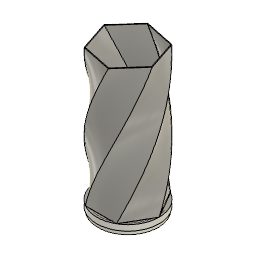
Assembly_lamp (Autodesk Fusion 360 archive; units mm, degrees)
design "hull_twisted"
part number: 2026-05-21-14-33-30-089
Autodesk Fusion 360 part; units mm, degrees
sketch "Sketch1" plane through (0, 0, 0) normal (0, 0, 1) x (1, 0, 0)
  circle A0 centre (0, 0) radius 38.75
  circle A1 centre (0, 0) radius 36.95
  dimension "d1" = 77.5
  dimension "d2" = 73.9
  constraint coincident A0.centre A1.centre
  constraint concentric A0 A1
  measures "d1" diameter of A0
  measures "d2" diameter of A1
extrude "Extrude1" add sketch "Sketch1" along normal blind 4.8 from surface at 17.9
sketch "Sketch2" plane through (0, 0, 22.7) normal (0, 0, 1) x (-1, 0, 0)
  circle A0 centre (0, 0) radius 36.95
  circle A1 centre (0, 0) radius 38.75
  circle A2 centre (0, 0) radius 40
  dimension "d6" = 80
  constraint coincident A0.centre A1.centre
  measures "d6" diameter of A2
extrude "Extrude2" add sketch "Sketch2" along normal blind 7.3 contours A1 | A2
sketch "Sketch3" plane through (0, 0, 30) normal (0, 0, 1) x (-1, 0, 0)
  circle A0 centre (0, 0) radius 36.95
  circle A1 centre (0, 0) radius 40
  line L0 (-20, 34.641) -> (-40, 0)
  line L1 (-40, 0) -> (-20, -34.641)
  line L2 (-20, -34.641) -> (20, -34.641)
  line L3 (20, -34.641) -> (40, 0)
  line L4 (40, 0) -> (20, 34.641)
  line L5 (20, 34.641) -> (-20, 34.641)
  line L6 (38.8453, 0) -> (19.4226, 33.641)
  line L7 (19.4226, 33.641) -> (-19.4226, 33.641)
  line L8 (-19.4226, 33.641) -> (-38.8453, 0)
  line L9 (-38.8453, 0) -> (-19.4226, -33.641)
  line L10 (-19.4226, -33.641) -> (19.4226, -33.641)
  line L11 (19.4226, -33.641) -> (38.8453, 0)
  dimension "d9" = 40
  dimension "d10" = -1
  constraint coincident A0.centre A1.centre
  constraint horizontal L3.end A0.centre
  measures "d9" distance of L0.start A0.centre
sketch "Sketch4" plane through (0, 0, 0) normal (0, 1, 0) x (1, 0, 0)
  line L0 (0, -30) -> (0, -200)
  dimension "d11" = 170
  constraint vertical L0
  measures "d11" distance of L0.start L0.end
sweep "Sweep1" add twist angle 108.3 profiles "Sketch3" path "Sketch4" along L0 section 1 contours A0 L4 L6 | A0 L3 L4 L6 L11 | A0 L3 L11 | A0 L4 L5 L6 L7 | A0 L2 L3 L10 L11 | A0 L5 L7 | A0 L2 L10 | A0 L0 L5 L7 L8 | A0 L1 L2 L9 L10 | A0 L0 L8 | A0 L1 L9 | A0 L0 L1 L8 L9
sketch "Sketch5" plane through (0, 0, 30) normal (0, 0, 1) x (-1, 0, 0)
  line L0 (-20, -34.641) -> (-23.5715, -28.455)
  arc A0 (-36.4285, -6.186) -> (-23.5715, -28.455) centre (0, 0) ccw
  line L1 (-36.4285, -6.186) -> (-40, 0)
  arc A1 (-40, 0) -> (-20, -34.641) centre (0, 0) ccw
  arc A2 (-36.4285, -6.186) -> (-23.5715, -28.455) centre (0, 0) ccw
  line L2 (-36.4285, -6.186) -> (-23.5715, -28.455)
extrude "Extrude3" add sketch "Sketch5" against normal blind 0.8 contours A0 A2 L2
pattern_circular "C-Pattern1" count 6 over 360 about axis through (0, 0, 1.75) along (0, 0, 1) of "Extrude3"

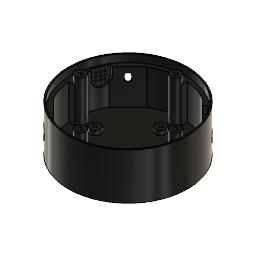
design "LAMP - BASE"
part number: 2026-05-21-10-57-22-259
Autodesk Fusion 360 part; units mm, degrees
sketch "Sketch1" plane through (0, 0, 0) normal (0, 0, 1) x (1, 0, 0)
  circle A0 centre (0, 0) radius 40
  circle A1 centre (0, 0) radius 39
  dimension "d1" = 80
  dimension "d2" = 78
  constraint coincident A0.centre A1.centre
  measures "d1" diameter of A0
  measures "d2" diameter of A1
extrude "Extrude1" add sketch "Sketch1" along normal blind 31
sketch "Sketch2" plane through (0, 0, 0) normal (0, 0, 1) x (1, 0, 0)
  circle A0 centre (0, 0) radius 39
  circle A1 centre (0, 0) radius 36.5
  dimension "d5" = 78
  dimension "d6" = 73
  constraint coincident A0.centre A1.centre
  constraint concentric A0 A1
  measures "d5" diameter of A0
  measures "d6" diameter of A1
extrude "Extrude2" add sketch "Sketch2" along normal blind 2.5 contours A0 | A1
extrude "Extrude3" add sketch "Sketch2" along normal blind 26
sketch "Sketch3" plane through (0, 0, 2.5) normal (0, 0, 1) x (-1, 0, 0)
  circle A0 centre (0, 0) radius 36.5
  circle A1 centre (0, 22) radius 3.5
  circle A2 centre (0, 22) radius 1.25
  circle A3 centre (-22, 0) radius 3.5
  circle A4 centre (-22, 0) radius 1.25
  circle A5 centre (0, -22) radius 3.5
  circle A6 centre (0, -22) radius 1.25
  circle A7 centre (22, 0) radius 3.5
  circle A8 centre (22, 0) radius 1.25
  dimension "d11" = 7
  dimension "d12" = 2.5
  dimension "d13" = 22
  dimension "d15" = 360
  constraint concentric A1 A2
  constraint vertical A0.centre A1.centre
  measures "d11" diameter of A1
  measures "d12" diameter of A2
  measures "d13" distance of A0.centre A1.centre
extrude "Extrude4" add sketch "Sketch3" along normal blind 3 contours A1 | A3 | A5 | A7
sketch "Sketch4" plane through (0, 0, 2.5) normal (0, 0, 1) x (-1, 0, 0)
  circle A0 centre (0, -22) radius 3.5
  circle A1 centre (-22, 0) radius 3.5
  circle A2 centre (0, 0) radius 36.5
  circle A3 centre (22, 0) radius 3.5
  circle A4 centre (0, 22) radius 3.5
  circle A5 centre (0, 32) radius 3.5
  circle A6 centre (0, 32) radius 1.25
  circle A7 centre (0, 0) radius 36.5
  line L0 (-3.5, 32) -> (-3.5, 36.3318)
  line L1 (3.5, 32) -> (3.5, 36.3318)
  dimension "d18" = 7
  dimension "d19" = 2.5
  dimension "d20" = 32
  constraint concentric A5 A6
  constraint vertical A2.centre A5.centre
  constraint coincident A5 L0.start
  constraint coincident A2 L0.end
  constraint tangent A5 L0
  constraint vertical L0
  constraint coincident A5 L1.start
  constraint coincident A2 L1.end
  constraint tangent A5 L1
  constraint parallel L0 L1
  measures "d18" diameter of A5
  measures "d19" diameter of A6
  measures "d20" vertical distance of A2.centre A5.centre
extrude "Extrude5" add sketch "Sketch4" along normal blind 28.5 contours A5
extrude "Extrude6" add sketch "Sketch4" along normal blind 23.5 contours A2 A5 A7 L0 L1 picked at (-2.1394, 35.9481)
pattern_circular "C-Pattern1" count 4 over 360 about axis through (0, 0, 1.75) along (0, 0, 1) of "Extrude5", "Extrude6"
sketch "Sketch5" plane through (0, 0, 26) normal (0, 0, 1) x (-1, 0, 0)
  arc A0 (36.3318, 3.5) -> (3.5, 36.3318) centre (0, 0) ccw
  circle A1 centre (0, 0) radius 39
  arc A2 (3.5, -36.3318) -> (36.3318, -3.5) centre (0, 0) ccw
  arc A3 (-36.3318, -3.5) -> (-3.5, -36.3318) centre (0, 0) ccw
  arc A4 (-3.5, 36.3318) -> (-36.3318, 3.5) centre (0, 0) ccw
  arc A5 (36.3318, 3.5) -> (3.5, 36.3318) centre (0, 0) ccw
  line L0 (31.3167, -18.7487) -> (18.7432, -31.32)
  line L1 (0, 0) -> (0, -13.7257) construction
  line L2 (0, 0) -> (13.0082, 0) construction
  line L3 (-31.3167, -18.7487) -> (-18.7432, -31.32)
  line L4 (31.3167, 18.7487) -> (18.7432, 31.32)
  line L5 (36.3318, 3.5) -> (32, 3.5)
  arc A6 (32, -3.5) -> (32, 3.5) centre (32, 0) ccw
  line L6 (32, -3.5) -> (36.3318, -3.5)
  arc A7 (3.5, -36.3318) -> (36.3318, -3.5) centre (0, 0) ccw
  line L7 (3.5, -36.3318) -> (3.5, -32)
  arc A8 (-3.5, -32) -> (3.5, -32) centre (0, -32) ccw
  line L8 (-3.5, -32) -> (-3.5, -36.3318)
  arc A9 (-36.3318, -3.5) -> (-3.5, -36.3318) centre (0, 0) ccw
  line L9 (-36.3318, -3.5) -> (-32, -3.5)
  arc A10 (-32, 3.5) -> (-32, -3.5) centre (-32, 0) ccw
  line L10 (-32, 3.5) -> (-36.3318, 3.5)
  arc A11 (-3.5, 36.3318) -> (-36.3318, 3.5) centre (0, 0) ccw
  line L11 (-3.5, 36.3318) -> (-3.5, 32)
  arc A12 (3.5, 32) -> (-3.5, 32) centre (0, 32) ccw
  line L12 (3.5, 32) -> (3.5, 36.3318)
  dimension "d27" = 17.78
  dimension "d28" = 16.046
  constraint coincident A0.centre A1.centre
  constraint vertical L1
  constraint perpendicular L1 L2
  constraint symmetric L0.start L1 L3.start
  constraint symmetric L0.end L1 L3.end
  constraint symmetric L0.start L2 L4.start
  constraint symmetric L0.end L2 L4.end
  measures "d27" distance of L0.start L0.end
  measures "d28" distance of A2.start L0.end
extrude "Extrude7" add sketch "Sketch5" against normal blind 23.5 contours A0 A5 L4 | A2 L0 A7 | A3 L3 A9
sketch "Sketch6" plane through (-25.03, -25.0344, 0) normal (0.707045, 0.707169, 0) x (-0.707169, 0.707045, 0)
  line L0 (-8.89, 2.5) -> (8.89, 2.5)
  line L1 (8.89, 2.5) -> (8.89, 26)
  line L2 (8.89, 26) -> (-8.89, 26)
  line L3 (-8.89, 26) -> (-8.89, 2.5)
  circle A0 centre (0, 13.5) radius 4.5
  dimension "d31" = 9
  dimension "d32" = 13.5
  constraint vertical origin A0.centre
  measures "d31" diameter of A0
  measures "d32" distance of origin A0.centre
extrude "Extrude8" cut sketch "Sketch6" against normal through all contours A0
sketch "Sketch7" plane through (-25.03, 25.0344, 0) normal (0.707045, -0.707169, 0) x (0.707169, 0.707045, 0)
  line L0 (-8.89, 2.5) -> (8.89, 2.5)
  line L1 (8.89, 2.5) -> (8.89, 26)
  line L2 (8.89, 26) -> (-8.89, 26)
  line L3 (-8.89, 26) -> (-8.89, 2.5)
  line L4 (-1.725, 21.025) -> (-1.725, 18.975)
  arc A0 (-1.725, 18.975) -> (1.725, 18.975) centre (0, 18.975) ccw
  line L5 (1.725, 18.975) -> (1.725, 21.025)
  arc A1 (1.725, 21.025) -> (-1.725, 21.025) centre (0, 21.025) ccw
  line L6 (0, 22.75) -> (0, 17.25) construction
  dimension "d34" = 3.45
  dimension "d35" = 5.5
  dimension "d36" = 14.75
  constraint tangent L4 A0
  constraint tangent A0 L5
  constraint parallel L4 L5
  constraint tangent L5 A1
  constraint tangent L4 A1
  constraint coincident A1 L6.start
  constraint coincident A0 L6.end
  constraint coincident A0.centre L6
  constraint coincident A1.centre L6
  constraint vertical L6
  constraint vertical origin A0.centre
  measures "d34" distance of L4 L5
  measures "d35" distance of L6.start L6.end
  measures "d36" distance of L0 L6.end
extrude "Extrude9" cut sketch "Sketch7" against normal blind 0.698 contours L4 A0 L5 A1
extrude "Extrude10" cut sketch "Sketch7" against normal through all draft 37 from surface at -0.698 contours L4 A0 L5 A1
sketch "Sketch8" plane through (25.03, 25.0344, 0) normal (-0.707045, -0.707169, 0) x (0.707169, -0.707045, 0)
  line L0 (8.89, 26) -> (-8.89, 26)
  line L1 (-8.89, 26) -> (-8.89, 2.5)
  line L2 (-8.89, 2.5) -> (8.89, 2.5)
  line L3 (8.89, 2.5) -> (8.89, 26)
  circle A0 centre (0, 11) radius 3.5
  line L4 (-3.5, 26) -> (-3.5, 11)
  line L5 (3.5, 26) -> (3.5, 11)
  dimension "d41" = 7
  dimension "d42" = 11
  constraint vertical origin A0.centre
  constraint coincident L0 L4.start
  constraint perpendicular L0 L4
  constraint coincident L0 L5.start
  constraint coincident A0 L5.end
  constraint coincident A0 L4.end
  constraint tangent A0 L4
  constraint tangent A0 L5
  constraint vertical L5
  measures "d41" diameter of A0
  measures "d42" vertical distance of origin A0.centre
extrude "Extrude11" cut sketch "Sketch8" against normal blind 2.6 contours L0 A0 L4 L5 | A0
extrude "Extrude12" cut sketch "Sketch8" against normal blind 4.6 contours A0
sketch "Sketch9" plane through (0, 0, 26) normal (0, 0, 1) x (-1, 0, 0)
  circle A0 centre (0, 0) radius 39
  line L0 (-22.5549, -27.509) -> (-24.3932, -29.3477)
  line L1 (-24.3932, -29.3477) -> (-29.3434, -24.3983)
  line L2 (-29.3434, -24.3983) -> (-27.505, -22.5597)
  line L3 (-27.505, -22.5597) -> (-31.3167, -18.7487)
  arc A1 (-36.3318, -3.5) -> (-31.3167, -18.7487) centre (0, 0) ccw
  line L4 (-36.3318, -3.5) -> (-32, -3.5)
  arc A2 (-32, 3.5) -> (-32, -3.5) centre (-32, 0) ccw
  line L5 (-32, 3.5) -> (-36.3318, 3.5)
  arc A3 (-3.5, 36.3318) -> (-36.3318, 3.5) centre (0, 0) ccw
  line L6 (-3.5, 36.3318) -> (-3.5, 32)
  arc A4 (3.5, 32) -> (-3.5, 32) centre (0, 32) ccw
  line L7 (3.5, 32) -> (3.5, 36.3318)
  arc A5 (18.7432, 31.32) -> (3.5, 36.3318) centre (0, 0) ccw
  line L8 (18.7432, 31.32) -> (31.3167, 18.7487)
  arc A6 (36.3318, 3.5) -> (31.3167, 18.7487) centre (0, 0) ccw
  line L9 (36.3318, 3.5) -> (32, 3.5)
  arc A7 (32, -3.5) -> (32, 3.5) centre (32, 0) ccw
  line L10 (32, -3.5) -> (36.3318, -3.5)
  arc A8 (31.3167, -18.7487) -> (36.3318, -3.5) centre (0, 0) ccw
  line L11 (31.3167, -18.7487) -> (18.7432, -31.32)
  arc A9 (3.5, -36.3318) -> (18.7432, -31.32) centre (0, 0) ccw
  line L12 (3.5, -36.3318) -> (3.5, -32)
  arc A10 (-3.5, -32) -> (3.5, -32) centre (0, -32) ccw
  line L13 (-3.5, -32) -> (-3.5, -36.3318)
  arc A11 (-18.7432, -31.32) -> (-3.5, -36.3318) centre (0, 0) ccw
  line L14 (-18.7432, -31.32) -> (-22.5549, -27.509)
  line L15 (31.3167, -18.7487) -> (18.7432, -31.32)
  arc A12 (31.3167, -18.7487) -> (36.3318, -3.5) centre (0, 0) ccw
  arc A13 (3.5, -36.3318) -> (18.7432, -31.32) centre (0, 0) ccw
  line L16 (36.4457, -10.9357) -> (32.1385, -20.5117)
  line L17 (32.1385, -20.5117) -> (30.3555, -19.7097)
  line L18 (36.4457, -10.9357) -> (35.0184, -10.2938)
  dimension "d50" = 10.5
  dimension "d51" = 17.212
  dimension "d52" = 1.565
  dimension "d53" = 1.955
  constraint coincident L15 L17.end
  constraint perpendicular L16 L17
  constraint coincident A8 L18.end
  constraint perpendicular L16 L18
  measures "d50" distance of L16.start L16.end
  measures "d51" distance of L11.end L16.end
  measures "d52" distance of L16.start L18.end
  measures "d53" distance of L16.end L17.end
extrude "Extrude13" cut sketch "Sketch9" against normal blind 5.8 contours A8 L11 L15 A12 L16 L17 L18
ref_plane "WorkPlane1" through (-30.3555, 19.7097, 26) normal (0.938263, -0.345923, 0) x (0.345923, 0.938263, 0)
sketch "Sketch10" plane through (-33.1202, 12.2109, 0) normal (0.938263, -0.345923, 0) x (0.345923, 0.938263, 0)
  line L0 (-2.4554, 20.2) -> (-2.4554, 26)
  line L1 (6.7581, 20.2) -> (-2.4554, 20.2)
  line L2 (7.9922, 20.2) -> (6.7581, 20.2)
  line L3 (7.9922, 26) -> (7.9922, 20.2)
  arc A0 (-2.4554, 20.2) -> (7.9922, 20.2) centre (2.7684, 20.2) ccw
  constraint tangent L3 A0
extrude "Extrude14" cut sketch "Sketch10" along normal up to surface end surface through (-36.4457, 10.9357, 26) normal (0.911992, -0.410207, 0) offset 0
sketch "Sketch11" plane through (-34.4041, 15.4747, 0) normal (0.911992, -0.410207, 0) x (0.410207, 0.911992, 0)
  line L0 (5.523, 26) -> (-4.977, 26)
  line L1 (-4.977, 26) -> (-4.977, 20.2)
  line L2 (-4.977, 20.2) -> (-5.0858, 20.2)
  ellipse E0 centre (0.1506, 20.2) end of major axis (-5.0858, 20.2) minor radius 5.2238 (-5.0858, 20.2) -> (5.387, 20.2) ccw
  line L3 (5.387, 20.2) -> (5.523, 20.2)
  line L4 (5.523, 20.2) -> (5.523, 26)
  circle A0 centre (2.622, 23.4) radius 0.6
  circle A1 centre (0.304, 23.4) radius 0.6
  circle A2 centre (-2.014, 23.4) radius 0.6
  circle A3 centre (2.622, 20.9) radius 0.6
  circle A4 centre (0.304, 20.9) radius 0.6
  circle A5 centre (-2.014, 20.9) radius 0.6
  circle A6 centre (2.622, 18.4) radius 0.6
  circle A7 centre (0.304, 18.4) radius 0.6
  circle A8 centre (-2.014, 18.4) radius 0.6
  dimension "d59" = 1.2
  dimension "d60" = 2.6
  dimension "d61" = 2.901
  dimension "d62" = 1.2
  dimension "d63" = 1.2
  dimension "d64" = 2.318
  dimension "d65" = 2.318
  dimension "d68" = 0
  dimension "d69" = -5
  constraint horizontal A0.centre A1.centre
  constraint horizontal A1.centre A2.centre
  measures "d59" diameter of A0
  measures "d60" distance of L0 A0.centre
  measures "d61" distance of L4 A0.centre
  measures "d62" diameter of A1
  measures "d63" diameter of A2
  measures "d64" distance of A0.centre A1.centre
  measures "d65" distance of A1.centre A2.centre
extrude "Extrude15" cut sketch "Sketch11" against normal through all contours A0 | A1 | A2 | A3 | A4 | A5 | A6 | A7 | A8
equation "d9 = 23.5 mm + 2.5 mm"

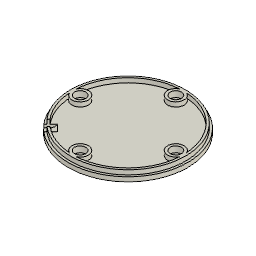
design "Top_cover"
part number: 2026-05-20-15-10-24-517
Autodesk Fusion 360 part; units mm, degrees
sketch "Sketch1" plane through (0, 0, 0) normal (0, 0, 1) x (1, 0, 0)
  circle A0 centre (0, 0) radius 40
  circle A1 centre (0, 0) radius 38.5
  dimension "d1" = 80
  dimension "d2" = 77
  constraint coincident A0.centre A1.centre
  constraint concentric A0 A1
  measures "d1" diameter of A0
  measures "d2" diameter of A1
extrude "Extrude1" add sketch "Sketch1" along normal blind 3 contours A0 | A1
extrude "Extrude2" add sketch "Sketch1" along normal blind 3 from surface at 3 contours A1
sketch "Sketch2" plane through (0, 0, 6) normal (0, 0, 1) x (-1, 0, 0)
  circle A0 centre (0, 0) radius 38.5
  circle A1 centre (0, 0) radius 37
  dimension "d8" = 74
  constraint coincident A0.centre A1.centre
  measures "d8" diameter of A1
extrude "Extrude3" cut sketch "Sketch2" against normal blind 3 contours A1
ref_plane "WorkPlane3" through (0, 0, 0) normal (-0.707107, 0.707107, 0) x (0, 0, 1)
sketch "Sketch3" plane through (0, 0, 0) normal (-0.707107, 0.707107, 0) x (0.707107, 0.707107, 0)
  line L0 (-38.5, -6) -> (38.5, -6)
  line L1 (38.5, -3) -> (-38.5, -3)
  line L2 (-40, -3) -> (40, -3)
  line L3 (-40, 0) -> (40, 0)
  line L4 (-40, -3) -> (-40, -1)
  line L5 (-40, -1) -> (-36.546, -1)
  line L6 (-40, -3) -> (-33.385, -3)
  arc A0 (-33.385, -3) -> (-36.546, -1) centre (-36.7574, -4.8322) ccw
  line L7 (-38.5, -6) -> (-36.5, -6)
  line L8 (-36.5, -6) -> (-36.5, -3)
  line L9 (-36.5, -3) -> (-38.5, -3)
  line L10 (-38.5, -3) -> (-38.5, -6)
  dimension "d11" = 2
  dimension "d12" = 3.454
  dimension "d13" = 6.615
  dimension "d14" = 3.838
  dimension "d15" = 3
  dimension "d16" = 2
  constraint coincident L2.start L4.start
  constraint perpendicular L2 L4
  constraint perpendicular L4 L5
  constraint perpendicular L4 L6
  constraint horizontal L7
  constraint vertical L8
  constraint horizontal L9
  constraint vertical L10
  constraint coincident L1.end L9.end
  measures "d11" distance of L2.start L4.end
  measures "d12" distance of L4.end L5.end
  measures "d13" distance of L2.start L6.end
  measures "d14" radius of A0
  measures "d15" distance of L0.start L1.end
  measures "d16" distance of L0.start L7.end
extrude "Extrude4" cut sketch "Sketch3" along normal mid plane 6
sketch "Sketch4" plane through (0, 0, 6) normal (0, 0, 1) x (-1, 0, 0)
  line L0 (23.9555, 28.1981) -> (25.0195, 29.2622)
  arc A0 (25.0195, 29.2622) -> (29.2622, 25.0195) centre (0, 0) ccw
  line L1 (29.2622, 25.0195) -> (28.1981, 23.9555)
  arc A1 (23.9555, 28.1981) -> (28.1981, 23.9555) centre (0, 0) ccw
  arc A2 (23.9555, 28.1981) -> (28.1981, 23.9555) centre (0, 0) ccw
  circle A3 centre (0, -32) radius 5.5
  circle A4 centre (0, -32) radius 3.75
  dimension "d19" = 11
  dimension "d20" = 7.5
  dimension "d23" = 32
  constraint vertical A0.centre A3.centre
  constraint concentric A3 A4
  measures "d19" diameter of A3
  measures "d20" diameter of A4
  measures "d23" distance of A0.centre A3.centre
extrude "Extrude5" add sketch "Sketch4" against normal blind 3 contours A1 A2 A3 | A1 A2 A3 | A4
extrude "Extrude6" cut sketch "Sketch4" against normal blind 4 contours A4
sketch "Sketch5" plane through (0, 0, 0) normal (0, 0, -1) x (1, 0, 0)
  circle A0 centre (0, 0) radius 40
  circle A1 centre (0, -32) radius 3.75
  circle A2 centre (0, -32) radius 3
  dimension "d26" = 6
  constraint concentric A1 A2
  measures "d26" diameter of A2
ref_plane "WorkPlane1" through (0, 0, 2) normal (0, 0, -1) x (1, 0, 0)
sketch "Sketch6" plane through (0, 0, 2) normal (0, 0, -1) x (-1, 0, 0)
  circle A0 centre (0, 32) radius 1.6
  point P0 (0, 32)
  dimension "d29" = 3.2
  constraint vertical P0 A0.centre
  constraint coincident P0 A0.centre
  measures "d29" diameter of A0
loft "Loft1" cut profiles "Sketch5", "Sketch6" section 1 contours A2 section 2
pattern_circular "C-Pattern1" count 4 over 360 about axis through (0, 0, 1.75) along (0, 0, 1) of "Extrude5", "Extrude6", "Loft1"
move_body "Move1" [suppressed]
equation "d2 = ( 38.5 * 2 ) * 1 mm"
equation "d8 = ( 37 * 2 ) * 1 mm"

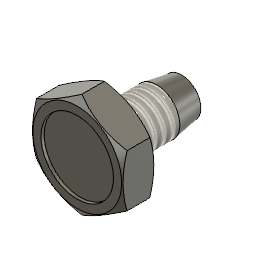
design "Large Indented Hex Head Tapping Screw ANSI B18.6.4 8-32 UNC x 0.25 Type C Steel Grade 2 Plain"
description: Large Indented Hex Head Tapping Screw ANSI B18.6.4 8-32 UNC x 0.25 Type C
part number: LIHHTSTC ANSI B18.6.4 - 8-32 UNC x 0.25 Steel Grade 2 Plain
Autodesk Fusion 360 part; units mm, degrees
sketch "Sketch1" plane through (0, 0, 0) normal (0, 1, 0) x (1, 0, 0)
  line L0 (0, 6.35) -> (0, -2.5146)
  line L1 (4.5766, -0.4003) -> (4.5766, -2.3937)
  line L2 (4.5766, -2.3937) -> (3.8832, -2.794)
  line L3 (3.8832, -2.794) -> (3.1699, -2.794)
  line L4 (2.0828, 0) -> (2.0828, 6.35)
  line L5 (2.0828, 6.35) -> (0, 6.35)
  line L6 (4.5766, -0.4003) -> (3.8832, 0)
  line L7 (3.8832, 0) -> (2.0828, 0)
  line L8 (3.1699, -2.794) -> (3.1699, -2.5146)
  line L9 (3.1699, -2.5146) -> (0, -2.5146)
  dimension "d6" = 30
  dimension "d9" = 9.1531
  dimension "d27" = 30
  dimension "d28" = 2.794
  dimension "d50" = 4.1656
  dimension "d54" = 6.3398
  dimension "d56" = 7.7663
  dimension "d59" = 0.2794
  dimension "d60" = 6.35
  constraint vertical L0
  constraint perpendicular L4 L7
  constraint coincident L0.start L5.end
  constraint coincident origin L0
  constraint coincident origin L7
  constraint perpendicular L0 L5
  constraint perpendicular L3 L8
  constraint coincident L0 L9.end
  constraint perpendicular L0 L9
  constraint coincident L0.end L9.end
  constraint vertical L2.end L6.end
  measures "d6" angle of L2 L3
  measures "d27" angle of L6 L7
  measures "d28" distance of L3 L7
  measures "d59" distance of L3.end L9
  measures "d60" distance of L4.start L5
revolve "Revolve1" add sketch "Sketch1" angle 360 about axis through (0, 0, 1.75) along (0, 0, 1)
sketch "Sketch2" plane through (0, 0, 2.794) normal (0, 0, 1) x (1, 0, 0)
  line L0 (-3.9624, -2.2877) -> (0, -4.5754)
  line L1 (0, -4.5754) -> (3.9624, -2.2877)
  line L2 (3.9624, -2.2877) -> (3.9624, 2.2877)
  line L3 (3.9624, 2.2877) -> (0, 4.5754)
  line L4 (0, 4.5754) -> (-3.9624, 2.2877)
  line L5 (-3.9624, 2.2877) -> (-3.9624, -2.2877)
  circle A0 centre (0, 0) radius 4.5964
  dimension "d65" = 7.9248
  dimension "d66" = 9.1928
  constraint coincident A0.centre origin
  constraint vertical L5
  measures "d65" distance of L2 L5
  measures "d66" diameter of A0
extrude "Extrude1" cut sketch "Sketch2" against normal blind 2.794
thread "Thread1" "ANSI Unified Screw Threads 0.164(#8) 8-32 UNC 8-32 UNC 2A" major diameter 4.0665 minor diameter 3.1979 pitch 0.7937 angle 60 resizes the face on face at (2.0802, -0.1038, -4.2333)
sketch "Sketch5" plane through (0, 0, 0) normal (0, 1, 0) x (1, 0, 0)
  line L0 (0, 0) -> (0, 6.35)
  line L1 (0, 6.35) -> (-2.1245, 6.35)
  line L2 (-2.1245, 6.35) -> (-2.1245, 3.5814)
  line L3 (-2.1245, 3.5814) -> (-1.6764, 6.35)
  point P0 (0, 6.35)
  dimension "d62" = 2.7686
  dimension "d63" = 1.6764
  dimension "d64" = 2.1245
  constraint perpendicular L0 L1
  constraint perpendicular L1 L2
  constraint coincident L1 L3.end
  constraint coincident P0 L0.end
  constraint vertical L0
  measures "d62" distance of L1 L2.end
  measures "d63" distance of L0 L3.end
  measures "d64" distance of L0 L1.end
revolve "Revolve2" cut sketch "Sketch5" angle 360 about axis through (0, 0, 1.75) along (0, 0, 1)
equation "d9 = adsk_headdia"
equation "d16 = -adsk_headh"
equation "d28 = adsk_headh"
equation "adsk_nomdia = 0.164 in"
equation "adsk_nomlen = 0.25 in"
equation "adsk_headdia = 0.36036 in"
equation "adsk_waflat = 0.312 in"
equation "adsk_headh = 0.11 in"
equation "adsk_indentdia = 0.2496 in"
equation "adsk_indentdepth = 0.011 in"
equation "adsk_endpointdia = 0.132 in"
equation "d50 = adsk_nomdia"
equation "adsk_startlen = 0.109 in"
equation "d54 = adsk_indentdia"
equation "adsk_beardia = adsk_waflat * 0.98"
equation "d56 = adsk_beardia"
equation "d59 = adsk_indentdepth"
equation "d60 = adsk_nomlen"
equation "d62 = adsk_startlen"
equation "d63 = adsk_endpointdia / 2"
equation "d64 = adsk_nomdia * 0.51"
equation "d65 = adsk_waflat"
equation "d66 = max(adsk_waflat * 1.16; adsk_headdia)"

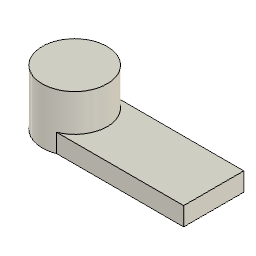
design "CAP-SCREW"
part number: 2026-05-20-21-13-29-780
Autodesk Fusion 360 part; units mm, degrees
sketch "Sketch1" plane through (0, 0, 0) normal (0, 0, 1) x (1, 0, 0)
  circle A0 centre (0, 0) radius 3.5
  line L0 (1.299, 3.25) -> (15, 3.25)
  line L1 (15, 3.25) -> (15, -3.25)
  line L2 (15, -3.25) -> (1.299, -3.25)
  line L3 (0, 0) -> (-14.556, 0) construction
  dimension "d1" = 7
  dimension "d2" = 13.701
  dimension "d3" = 6.5
  constraint coincident A0.centre L3.start
  constraint horizontal L0
  constraint vertical L1
  constraint horizontal L2
  constraint coincident A0 L0.start
  constraint horizontal L3
  constraint symmetric L0 L2 L3
  measures "d1" diameter of A0
  measures "d2" distance of L0.start L0.end
  measures "d3" distance of L0.end L1.end
extrude "Extrude1" add sketch "Sketch1" along normal blind 6 contours A0
extrude "Extrude2" add sketch "Sketch1" along normal blind 2 contours A0 L0 L1 L2

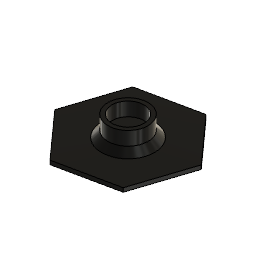
design "twisted top"
part number: 2026-05-21-00-01-04-472
Autodesk Fusion 360 part; units mm, degrees
sketch "Sketch1" plane through (0, 0, 0) normal (0, 0, 1) x (1, 0, 0)
  line L0 (-25.748, 28.7303) -> (11.9841, 36.6874)
  line L1 (11.9841, 36.6874) -> (37.7548, 7.9326)
  line L2 (37.7548, 7.9326) -> (25.748, -28.7303)
  line L3 (25.748, -28.7303) -> (-11.9841, -36.6874)
  line L4 (-11.9841, -36.6874) -> (-37.7548, -7.9326)
  line L5 (-37.7548, -7.9326) -> (-25.748, 28.7303)
  line L6 (-25.748, 28.7303) -> (25.748, -28.7303) construction
  dimension "d1" = 38.562
  dimension "d2" = 38.562
  dimension "d3" = 38.613
  dimension "d4" = 38.613
  dimension "d5" = 38.579
  dimension "d6" = 38.579
  dimension "d7" = 66.85
  dimension "d8" = 66.82
  constraint parallel L0 L3
  constraint parallel L1 L4
  constraint midpoint origin L6
  measures "d1" distance of L0.start L0.end
  measures "d2" distance of L2.end L3.end
  measures "d3" distance of L0.end L1.end
  measures "d4" distance of L3.end L4.end
  measures "d5" distance of L1.end L2.end
  measures "d6" distance of L0.start L4.end
  measures "d7" distance of L0 L3
  measures "d8" distance of L1 L4
extrude "Extrude1" add sketch "Sketch1" along normal blind 2.5
sketch "Sketch2" plane through (0, 0, 2.5) normal (0, 0, 1) x (-1, 0, 0)
  line L0 (37.7548, 7.9326) -> (11.9841, 36.6874)
  line L1 (11.9841, 36.6874) -> (-25.748, 28.7303)
  line L2 (-25.748, 28.7303) -> (-37.7548, -7.9326)
  line L3 (-37.7548, -7.9326) -> (-11.9841, -36.6874)
  line L4 (-11.9841, -36.6874) -> (25.748, -28.7303)
  line L5 (25.748, -28.7303) -> (37.7548, 7.9326)
  circle A0 centre (0, 0) radius 16.5
  dimension "d11" = 33
  constraint coincident A0.centre origin
  measures "d11" diameter of A0
extrude "Extrude2" add sketch "Sketch2" along normal blind 4 draft -45 contours A0
sketch "Sketch3" plane through (0, 0, 6.5) normal (0, 0, 1) x (-1, 0, 0)
  circle A0 centre (0, 0) radius 12.5
  circle A1 centre (0, 0) radius 10
  circle A2 centre (0, 0) radius 12.5
  dimension "d14" = 20
  dimension "d15" = 25
  constraint coincident A0.centre A1.centre
  constraint concentric A1 A2
  measures "d14" diameter of A1
  measures "d15" diameter of A2
extrude "Extrude3" add sketch "Sketch3" along normal blind 8.5

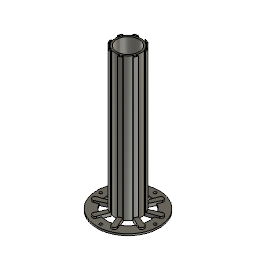
design "lamp_core by satwik"
part number: 2026-05-20-20-38-45-437
Autodesk Fusion 360 part; units mm, degrees
sketch "Sketch1" plane through (0, 0, 0) normal (0, 0, 1) x (1, 0, 0)
  circle A0 centre (0, 0) radius 15
  circle A1 centre (0, 0) radius 13
  dimension "d1" = 30
  dimension "d2" = 26
  constraint coincident A0.centre A1.centre
  measures "d1" diameter of A0
  measures "d2" diameter of A1
extrude "Extrude1" add sketch "Sketch1" along normal blind 168
sketch "Sketch2" plane through (0, 0, 168) normal (0, 0, 1) x (-1, 0, 0)
  circle A0 centre (0, 0) radius 13
  circle A1 centre (0, 0) radius 15
  circle A2 centre (0, 0) radius 15
  line L0 (0, 0) -> (0, -29.5553) construction
  line L1 (-4.979, -14.1495) -> (-5.3534, -15.1839)
  line L2 (-6.4858, -13.5253) -> (-6.9525, -14.5214)
  line L3 (-6.9525, -14.5214) -> (-8.3108, -13.8851)
  line L4 (-5.3534, -15.1839) -> (-3.943, -15.6944)
  line L5 (-8.3108, -13.8851) -> (-8.735, -14.7907)
  line L6 (-3.943, -15.6944) -> (-4.2834, -16.6347)
  arc A3 (-8.735, -14.7907) -> (-4.2834, -16.6347) centre (-0.0303, -0.0721) ccw
  line L7 (-6.4858, -13.5253) -> (-4.979, -14.1495)
  line L8 (-5.7324, -13.8374) -> (-8.1748, -19.7332)
  dimension "d5" = 19.9
  dimension "d6" = 25.1
  dimension "d7" = 1.1
  dimension "d8" = 1.1
  dimension "d9" = 1.5
  dimension "d10" = 1.5
  dimension "d11" = 1
  dimension "d12" = 1
  dimension "d16" = 1.631
  dimension "d17" = 3.943
  dimension "d18" = 25.1
  dimension "d19" = 17.1
  constraint coincident A0.centre A1.centre
  constraint vertical L0
  constraint coincident A2 L1.start
  constraint coincident A2 L2.start
  constraint perpendicular L1 L4
  constraint perpendicular L3 L5
  constraint perpendicular L4 L6
  constraint midpoint L7 L8.start
  constraint perpendicular L7 L8
  measures "d5" angle of L0 L1
  measures "d6" angle of L0 L2
  measures "d7" distance of L2.start L2.end
  measures "d8" distance of L1.start L1.end
  measures "d9" distance of L2.end L3.end
  measures "d10" distance of L1.end L4.end
  measures "d11" distance of L3.end L5.end
  measures "d12" distance of L4.end L6.end
  measures "d16" distance of L1.start L2.start
  measures "d17" distance of L0 L4.end
  measures "d18" angle of L0 L5
  measures "d19" radius of A3
extrude "Extrude2" add sketch "Sketch2" along normal blind 168 from surface at -168 contours A1 A2 L2 L3 L5 A3 L8 | A1 A2 L1 L4 L6 A3 L8
sketch "Sketch3" plane through (0, 0, 168) normal (0, 0, 1) x (-1, 0, 0)
  circle A0 centre (0, 0) radius 13
  arc A1 (-4.979, -14.1495) -> (-6.4858, -13.5253) centre (0, 0) ccw
  line L0 (-6.4858, -13.5253) -> (-6.9525, -14.5214)
  line L1 (-6.9525, -14.5214) -> (-8.3108, -13.8851)
  line L2 (-8.3108, -13.8851) -> (-8.735, -14.7907)
  arc A2 (-8.735, -14.7907) -> (-4.2834, -16.6347) centre (-0.0303, -0.0721) ccw
  line L3 (-4.2834, -16.6347) -> (-3.943, -15.6944)
  line L4 (-3.943, -15.6944) -> (-5.3534, -15.1839)
  line L5 (-5.3534, -15.1839) -> (-4.979, -14.1495)
  line L6 (-5.3534, -15.1839) -> (-3.943, -15.6944)
  line L7 (-3.943, -15.6944) -> (-8.6402, -28.6704)
  line L8 (-6.9525, -14.5214) -> (-8.3108, -13.8851)
  line L9 (-8.3108, -13.8851) -> (-14.1648, -26.382)
  arc A3 (-14.1648, -26.382) -> (-8.6402, -28.6704) centre (-11.3916, -27.4999) ccw
  line L10 (-5.3534, -15.1839) -> (-6.9525, -14.5214)
  dimension "d20" = 13.8
  dimension "d22" = 13.8
  dimension "d23" = 2.99
  constraint coincident L4.end L5.start
  constraint coincident L3.end L4.start
  constraint perpendicular L4 L7
  constraint coincident L0.end L1.start
  constraint coincident L1.end L2.start
  constraint perpendicular L1 L9
  measures "d20" distance of L1.end L9.end
  measures "d22" distance of L3.end L7.end
  measures "d23" radius of A3
extrude "Extrude3" add sketch "Sketch3" along normal blind 4 from surface at -168 contours L1 L2 A2 L3 L4 L6 L7 L8 L9 L10 | A2 L7 L9 A3
pattern_circular "C-Pattern1" count 8 over 360 about axis through (0, 0, 1.75) along (0, 0, 1) of "Extrude2", "Extrude3"
sketch "Sketch4" plane through (0, 0, 0) normal (0, 0, 1) x (1, 0, 0)
  circle A0 centre (0, 0) radius 36.6
  circle A1 centre (0, 0) radius 25
  dimension "d29" = 50
  dimension "d30" = 73.2
  constraint coincident A0.centre A1.centre
  constraint concentric A0 A1
  measures "d29" diameter of A1
  measures "d30" diameter of A0
extrude "Extrude4" add sketch "Sketch4" along normal blind 2
sketch "Sketch5" plane through (0, 0, 0) normal (0, 0, 1) x (1, 0, 0)
  circle A0 centre (0, 32) radius 1.6
  dimension "d33" = 3.2
  dimension "d34" = 32
  constraint vertical origin A0.centre
  measures "d33" diameter of A0
  measures "d34" vertical distance of origin A0.centre
extrude "Extrude5" cut sketch "Sketch5" along normal blind 2
pattern_circular "C-Pattern2" count 4 over 360 about axis through (0, 0, 1.75) along (0, 0, 1) of "Extrude5"
